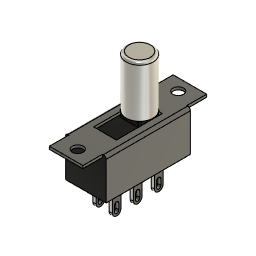
Diag_UP_SX64_PCB_v1 v6 (Autodesk Fusion 360 archive; units mm, degrees)
design "switch_slide_19mm"
Autodesk Fusion 360 part; units mm, degrees
sketch "Skizze1" plane through (0, 0, 0) normal (0, 0, 1) x (1, 0, 0)
  line L0 (3.1, 11.45) -> (-3.1, 11.45)
  line L1 (-3.1, 11.45) -> (-3.1, -11.45)
  line L2 (-3.1, -11.45) -> (3.1, -11.45)
  line L3 (3.1, -11.45) -> (3.1, 11.45)
  line L4 (3.1, 11.45) -> (-3.1, -11.45) construction
  line L5 (-3.1, 11.45) -> (3.1, -11.45) construction
  line L6 (3.75, 7.8) -> (-3.75, 7.8)
  line L7 (-3.75, 7.8) -> (-3.75, -7.8)
  line L8 (-3.75, -7.8) -> (3.75, -7.8)
  line L9 (3.75, -7.8) -> (3.75, 7.8)
  line L10 (3.75, 7.8) -> (-3.75, -7.8) construction
  line L11 (-3.75, 7.8) -> (3.75, -7.8) construction
  line L12 (0, 0) -> (6.5711, 0) construction
  line L13 (0, 0) -> (0, 13.796) construction
  line L14 (2.1, 4.25) -> (-2.1, 4.25)
  line L15 (-2.1, 4.25) -> (-2.1, -4.25)
  line L16 (-2.1, -4.25) -> (2.1, -4.25)
  line L17 (2.1, -4.25) -> (2.1, 4.25)
  line L18 (2.1, 4.25) -> (-2.1, -4.25) construction
  line L19 (-2.1, 4.25) -> (2.1, -4.25) construction
  line L20 (-1.6, 0.25) -> (1.6, 0.25)
  line L21 (1.9, 0.55) -> (1.9, 3.75)
  line L22 (1.6, 4.05) -> (-1.6, 4.05)
  line L23 (-1.9, 3.75) -> (-1.9, 0.55)
  arc A0 (-1.6, 4.05) -> (-1.9, 3.75) centre (-1.6, 3.75) ccw
  arc A1 (1.9, 3.75) -> (1.6, 4.05) centre (1.6, 3.75) ccw
  arc A2 (1.6, 0.25) -> (1.9, 0.55) centre (1.6, 0.55) ccw
  arc A3 (-1.9, 0.55) -> (-1.6, 0.25) centre (-1.6, 0.55) ccw
  line L24 (-1.9, 2.15) -> (1.9, 2.15) construction
  circle A4 centre (0, 2.15) radius 2.5
  circle A5 centre (0, 9.3) radius 1
  line L25 (0, 0) -> (0, -9.9922) construction
  circle A6 centre (0, -9.3) radius 1
  point P0 (1.9, 4.05)
  point P1 (-1.9, 4.05)
  dimension "d133" = 6.2
  dimension "d134" = 22.9
  dimension "d135" = 7.5
  dimension "d136" = 15.6
  dimension "d137" = 4.2
  dimension "d138" = 8.5
  dimension "d139" = 3.8
  dimension "d140" = 3.8
  dimension "d141" = 0.2
  dimension "d142" = 0.2
  dimension "d143" = 0.3
  dimension "d144" = 0.3
  dimension "d145" = 0.3
  dimension "d146" = 0.3
  dimension "d147" = 5
  dimension "d148" = 2
  dimension "d149" = 9.3
  constraint perpendicular L0 L1
  constraint parallel L0 L2
  constraint parallel L1 L3
  constraint horizontal L0
  constraint coincident L4 L12.start
  constraint coincident L5 L12.start
  constraint coincident L12.start L13.start
  constraint perpendicular L6 L7
  constraint parallel L6 L8
  constraint parallel L7 L9
  constraint horizontal L6
  constraint coincident L10 L12.start
  constraint coincident L11 L12.start
  constraint perpendicular L9 L12
  constraint perpendicular L0 L13
  constraint perpendicular L14 L15
  constraint parallel L14 L16
  constraint parallel L15 L17
  constraint horizontal L14
  constraint coincident L18 L12.start
  constraint coincident L19 L12.start
  constraint horizontal L20
  constraint vertical L21
  constraint horizontal L22
  constraint vertical L23
  constraint coincident P1 L22
  constraint coincident P1 L23
  constraint tangent L22 A0
  constraint tangent L23 A0
  constraint coincident P0 L22
  constraint coincident P0 L21
  constraint tangent L22 A1
  constraint tangent L21 A1
  constraint tangent L21 A2
  constraint tangent L20 A2
  constraint tangent L23 A3
  constraint tangent L20 A3
  constraint midpoint L23 L24.start
  constraint midpoint L21 L24.end
  constraint midpoint L24 A4.centre
  constraint coincident L13 A5.centre
  constraint perpendicular L8 L25
  constraint coincident L25 A6.centre
  constraint symmetric L12 A5 A6
  measures "d133" distance of L1.end L2.end
  measures "d134" distance of L0.end L1.end
  measures "d135" distance of L7.end L8.end
  measures "d136" distance of L6.end L7.end
  measures "d137" distance of L15.end L16.end
  measures "d138" distance of L14.end L15.end
  measures "d139" distance of P0 P1
  measures "d140" distance of L20 L22
  measures "d141" distance of L17 L21
  measures "d142" distance of L14 L22
  measures "d143" radius of A0
  measures "d144" radius of A1
  measures "d145" radius of A2
  measures "d146" radius of A3
  measures "d147" diameter of A4
  measures "d148" diameter of A5
  measures "d149" distance of L12.start A5.centre
extrude "Extrusion1" add sketch "Skizze1" against normal blind 0.5 contours L0 L1 L3 L6 | L1 L3 L6 L8 | L1 L2 L3 L8 | L14 A4 | L17 A4 | L15 A4
extrude "Extrusion2" add sketch "Skizze1" against normal blind 0.5 contours L3 L6 L8 L9 | L1 L6 L7 L8
extrude "Extrusion3" add sketch "Skizze1" against normal blind 7 from surface at -0.5 contours L3 L6 L8 L9 | L1 L3 L6 L8 | L1 L6 L7 L8 | L14 L17 A1 A4 | L14 L22 A0 A1 A4 | L14 A4 | L17 A4 | L17 L21 A1 A2 A4 | L14 L15 A0 A4 | L20 L21 L22 L23 A0 A1 A2 A3 A4 | A1 A4 | L15 L16 L17 A2 A3 A4 | A0 A4 | A2 A4 | L15 L23 A0 A3 A4 | L15 A4 | L20 A2 A3 A4 | A3 A4
fillet "Abrundung1" radius 0.5 2 edges at (3.75, 0, 0) (-3.75, 0, 0)
extrude "Extrusion4" add sketch "Skizze1" along normal blind 0.5 and the other way blind 0.5 contours L20 L21 L22 L23 A0 A1 A2 A3 A4 | A1 A4 | A0 A4 | A2 A4 | A3 A4
extrude "Extrusion5" add sketch "Skizze1" along normal blind 9.5 from surface at 0.5 contours L14 L22 A0 A1 A4 | L14 A4 | L17 A4 | L17 L21 A1 A2 A4 | L20 L21 L22 L23 A0 A1 A2 A3 A4 | L15 L23 A0 A3 A4 | L15 A4 | L20 A2 A3 A4
fillet "Abrundung2" radius 0.5 1 edges at (-2.3308, 1.246, 10)
sketch "Skizze2" plane through (0, 0, -7.5) normal (0, 0, -1) x (1, 0, 0)
  line L0 (3.75, -7.8) -> (3.75, 7.8)
  line L1 (3.75, 7.8) -> (-3.75, 7.8)
  line L2 (-3.75, 7.8) -> (-3.75, -7.8)
  line L3 (-3.75, -7.8) -> (3.75, -7.8)
  line L4 (3.75, 7.8) -> (3.75, -7.8)
  line L5 (-3.75, 7.8) -> (3.75, 7.8)
  line L6 (-3.75, -7.8) -> (-3.75, 7.8)
  line L7 (3.75, -7.8) -> (-3.75, -7.8)
  line L8 (0, 0) -> (0, 9.0857) construction
  line L9 (0, 0) -> (7.5179, 0) construction
  line L10 (1.2, 0.8) -> (1.8, 0.8)
  line L11 (1.8, 0.8) -> (1.8, -0.8)
  line L12 (1.8, -0.8) -> (1.2, -0.8)
  line L13 (1.2, -0.8) -> (1.2, 0.8)
  line L14 (-1.8, 0.8) -> (-1.2, 0.8)
  line L15 (-1.2, 0.8) -> (-1.2, -0.8)
  line L16 (-1.2, -0.8) -> (-1.8, -0.8)
  line L17 (-1.8, -0.8) -> (-1.8, 0.8)
  line L18 (1.2, 3.1) -> (1.8, 3.1)
  line L19 (1.8, 3.1) -> (1.8, 4.7)
  line L20 (1.8, 4.7) -> (1.2, 4.7)
  line L21 (1.2, 4.7) -> (1.2, 3.1)
  line L22 (-1.8, 4.7) -> (-1.2, 4.7)
  line L23 (-1.2, 4.7) -> (-1.2, 3.1)
  line L24 (-1.2, 3.1) -> (-1.8, 3.1)
  line L25 (-1.8, 3.1) -> (-1.8, 4.7)
  line L26 (1.2, -3.1) -> (1.8, -3.1)
  line L27 (1.8, -3.1) -> (1.8, -4.7)
  line L28 (1.8, -4.7) -> (1.2, -4.7)
  line L29 (1.2, -4.7) -> (1.2, -3.1)
  line L30 (-1.8, -3.1) -> (-1.2, -3.1)
  line L31 (-1.2, -3.1) -> (-1.2, -4.7)
  line L32 (-1.2, -4.7) -> (-1.8, -4.7)
  line L33 (-1.8, -4.7) -> (-1.8, -3.1)
  dimension "d166" = 0.6
  dimension "d167" = 1.6
  dimension "d168" = 1.2
  dimension "d169" = 1.6
  dimension "d170" = 5.5
  constraint coincident L8.start L9.start
  constraint perpendicular L1 L8
  constraint perpendicular L4 L9
  constraint horizontal L10
  constraint vertical L11
  constraint horizontal L12
  constraint vertical L13
  constraint symmetric L9 L10 L12
  constraint horizontal L14
  constraint vertical L15
  constraint horizontal L16
  constraint vertical L17
  constraint symmetric L8 L11 L17
  constraint symmetric L8 L10 L14
  constraint symmetric L8 L12 L16
  constraint symmetric L8 L13 L15
  constraint horizontal L18
  constraint vertical L19
  constraint horizontal L20
  constraint vertical L21
  constraint collinear L13 L21
  constraint collinear L11 L19
  constraint horizontal L22
  constraint vertical L23
  constraint horizontal L24
  constraint vertical L25
  constraint collinear L17 L25
  constraint collinear L15 L23
  constraint collinear L20 L22
  constraint collinear L18 L24
  constraint horizontal L26
  constraint vertical L27
  constraint horizontal L28
  constraint vertical L29
  constraint collinear L13 L29
  constraint collinear L11 L27
  constraint symmetric L9 L18 L26
  constraint symmetric L9 L20 L28
  constraint horizontal L30
  constraint vertical L31
  constraint horizontal L32
  constraint vertical L33
  constraint collinear L17 L33
  constraint collinear L15 L31
  constraint collinear L26 L30
  constraint collinear L28 L32
  measures "d166" distance of L10.start L10.end
  measures "d167" distance of L10.end L11.end
  measures "d168" distance of L8 L13
  measures "d169" distance of L18 L20
  measures "d170" distance of L12 L20
extrude "Extrusion6" add sketch "Skizze2" along normal blind 5 contours L10 L11 L12 L13 | L14 L15 L16 L17 | L18 L19 L20 L21 | L22 L23 L24 L25 | L26 L27 L28 L29 | L30 L31 L32 L33
fillet "Abrundung3" radius 0.8 12 edges at (-1.5, -3.1, -12.5) (-1.5, -4.7, -12.5) (1.5, -4.7, -12.5) (1.5, -3.1, -12.5) (-1.5, -0.8, -12.5) (-1.5, 0.8, -12.5) (1.5, 0.8, -12.5) (1.5, -0.8, -12.5) (-1.5, 4.7, -12.5) (-1.5, 3.1, -12.5) (1.5, 3.1, -12.5) (1.5, 4.7, -12.5)
sketch "Skizze3" plane through (-1.8, 0, 0) normal (-1, 0, 0) x (0, -1, 0)
  arc A0 (-0.8, -11.7) -> (0.8, -11.7) centre (0, -11.7) ccw
  line L0 (0.8, -11.7) -> (0.8, -7.5)
  line L1 (0.8, -7.5) -> (-0.8, -7.5)
  line L2 (-0.8, -7.5) -> (-0.8, -11.7)
  line L3 (-4.7, -7.5) -> (-4.7, -11.7)
  arc A1 (-4.7, -11.7) -> (-3.1, -11.7) centre (-3.9, -11.7) ccw
  line L4 (-3.1, -7.5) -> (-3.1, -11.7)
  line L5 (-0.8, -7.5) -> (-0.8, -11.7)
  arc A2 (-0.8, -11.7) -> (0.8, -11.7) centre (0, -11.7) ccw
  line L6 (0.8, -7.5) -> (0.8, -11.7)
  line L7 (3.1, -7.5) -> (3.1, -11.7)
  line L8 (4.7, -7.5) -> (4.7, -11.7)
  arc A3 (3.1, -11.7) -> (4.7, -11.7) centre (3.9, -11.7) ccw
  line L9 (4.7, -11.7) -> (4.7, -7.5)
  line L10 (4.7, -7.5) -> (3.1, -7.5)
  line L11 (3.1, -7.5) -> (3.1, -11.7)
  line L12 (7.8, -7.5) -> (-7.8, -7.5)
  line L13 (-4.3, -10.6) -> (-4.3, -11.7)
  arc A4 (-4.3, -11.7) -> (-3.5, -11.7) centre (-3.9, -11.7) ccw
  line L14 (-3.5, -10.6) -> (-3.5, -11.7)
  line L15 (-0.4, -10.6) -> (-0.4, -11.7)
  arc A5 (-0.4, -11.7) -> (0.4, -11.7) centre (0, -11.7) ccw
  line L16 (0.4, -11.7) -> (0.4, -10.6)
  line L17 (3.5, -10.6) -> (3.5, -11.7)
  arc A6 (3.5, -11.7) -> (4.3, -11.7) centre (3.9, -11.7) ccw
  line L18 (4.3, -11.7) -> (4.3, -10.6)
  line L19 (-3.9, -10.2) -> (-3.9, -10.2)
  line L20 (0, -10.2) -> (0, -10.2)
  line L21 (3.9, -10.2) -> (3.9, -10.2)
  arc A7 (0, -10.2) -> (-0.4, -10.6) centre (0, -10.6) ccw
  arc A8 (0.4, -10.6) -> (0, -10.2) centre (0, -10.6) ccw
  arc A9 (-3.5, -10.6) -> (-3.9, -10.2) centre (-3.9, -10.6) ccw
  arc A10 (-3.9, -10.2) -> (-4.3, -10.6) centre (-3.9, -10.6) ccw
  arc A11 (3.9, -10.2) -> (3.5, -10.6) centre (3.9, -10.6) ccw
  arc A12 (4.3, -10.6) -> (3.9, -10.2) centre (3.9, -10.6) ccw
  dimension "d178" = 0.4
  dimension "d179" = 0.4
  dimension "d180" = 0.4
  dimension "d181" = 0.4
  dimension "d182" = 0.4
  dimension "d183" = 0.4
  dimension "d184" = 0.4
  dimension "d185" = 1.1
  dimension "d186" = 0.4
  dimension "d187" = 0.4
  dimension "d188" = 1.1
  dimension "d189" = 1.1
  constraint parallel L3 L13
  constraint concentric A1 A4
  constraint parallel L4 L14
  constraint tangent L13 A4
  constraint tangent A4 L14
  constraint parallel L2 L15
  constraint concentric A0 A5
  constraint parallel L0 L16
  constraint tangent L15 A5
  constraint tangent A5 L16
  constraint parallel L7 L17
  constraint concentric A3 A6
  constraint parallel L9 L18
  constraint tangent L17 A6
  constraint tangent A6 L18
  constraint tangent L15 A7
  constraint tangent L16 A8
  constraint tangent L14 A9
  constraint tangent L13 A10
  constraint tangent L17 A11
  constraint tangent L18 A12
  constraint collinear A7.centre A9.centre A11.centre
  measures "d178" distance of L3 L13
  measures "d179" distance of L5 L15
  measures "d180" distance of L7 L17
  measures "d181" radius of A7
  measures "d182" radius of A8
  measures "d183" radius of A9
  measures "d184" radius of A10
  measures "d185" distance of A1.centre A9.centre
  measures "d186" radius of A11
  measures "d187" radius of A12
  measures "d188" distance of A0.centre A7.centre
  measures "d189" distance of A3.centre A11.centre
extrude "Extrusion7" cut sketch "Skizze3" against normal blind 4 contours L13 A4 L14 A9 A10 | L15 A5 L16 A7 A8 | L17 A6 L18 A11 A12
ref_plane "Arbeitsebene1" through (0, 0, -3.75) normal (1, 0, 0) x (0, -1, 0)
equation "d169 = d167"
named bodies: "switch"
